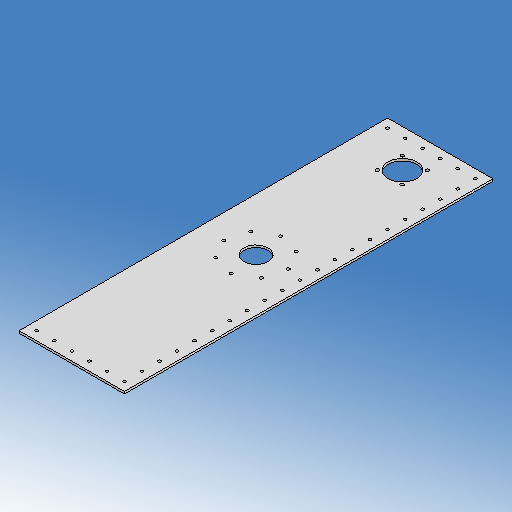
# Autodesk Inventor part: Armplate
Saved by Autodesk Inventor 2025 (Build 290162000, 162)
## iProperties
Created: 2024-06-23
Part Number: Armplate
Material: Generic
Document SubType Name: Modeling
Designer: seene
Density: 1 g/cm^3
Appearance: Default
Author: seene
Autodesk Inventor part; units mm, degrees
ref_plane "YZ Plane" through (0, 0, 0) normal (1, 0, 0) x (0, 1, 0)
ref_plane "XZ Plane" through (0, 0, 0) normal (0, 1, 0) x (-1, 0, 0)
ref_plane "XY Plane" through (0, 0, 0) normal (0, 0, 1) x (1, 0, 0)
sketch "Sketch1" plane through (0, 0, 0) normal (0, 1, 0) x (-1, 0, 0)
  line L0 (0, 0) -> (152.4, 0)
  line L1 (152.4, 0) -> (152.4, -533.4)
  line L2 (152.4, -533.4) -> (0, -533.4)
  line L3 (0, -533.4) -> (0, 0)
  circle A0 centre (76.2, -266.7) radius 47.25 construction
  circle A1 centre (76.2, -266.7) radius 41.5 construction
  circle A2 centre (76.2, -266.7) radius 17.5
  circle A3 centre (101.5192, -233.8186) radius 2.25
  circle A4 centre (70.8527, -225.5459) radius 2.25
  circle A5 centre (43.3186, -241.3808) radius 2.25
  circle A6 centre (35.0459, -272.0473) radius 2.25
  circle A7 centre (50.8808, -299.5814) radius 2.25
  circle A8 centre (81.5473, -307.8541) radius 2.25
  circle A9 centre (109.0814, -292.0192) radius 2.25
  circle A10 centre (117.3541, -261.3527) radius 2.25
  circle A11 centre (139.7, -12.7) radius 2.0701
  line L4 (152.4, -24.6076) -> (0, -26.1951) construction
  line L5 (152.4, -266.7) -> (0, -266.7) construction
  circle A12 centre (139.7, -520.7) radius 2.0701
  line L6 (152.4, -508.7924) -> (0, -507.2049) construction
  circle A13 centre (114.3, -12.7) radius 2.0701
  circle A14 centre (114.3, -520.7) radius 2.0701
  circle A15 centre (88.9, -12.7) radius 2.0701
  circle A16 centre (88.9, -520.7) radius 2.0701
  circle A17 centre (63.5, -12.7) radius 2.0701
  circle A18 centre (63.5, -520.7) radius 2.0701
  circle A19 centre (38.1, -12.7) radius 2.0701
  circle A20 centre (38.1, -520.7) radius 2.0701
  circle A21 centre (12.7, -12.7) radius 2.0701
  circle A22 centre (12.7, -520.7) radius 2.0701
  circle A23 centre (12.7, -38.1) radius 2.0701
  circle A24 centre (12.7, -63.5) radius 2.0701
  circle A25 centre (12.7, -88.9) radius 2.0701
  circle A26 centre (12.7, -114.3) radius 2.0701
  circle A27 centre (12.7, -139.7) radius 2.0701
  circle A28 centre (12.7, -165.1) radius 2.0701
  circle A29 centre (12.7, -190.5) radius 2.0701
  circle A30 centre (12.7, -215.9) radius 2.0701
  circle A31 centre (12.7, -241.3) radius 2.0701
  circle A32 centre (12.7, -266.7) radius 2.0701
  circle A33 centre (12.7, -292.1) radius 2.0701
  circle A34 centre (12.7, -317.5) radius 2.0701
  circle A35 centre (12.7, -342.9) radius 2.0701
  circle A36 centre (12.7, -368.3) radius 2.0701
  circle A37 centre (12.7, -393.7) radius 2.0701
  circle A38 centre (12.7, -419.1) radius 2.0701
  circle A39 centre (12.7, -444.5) radius 2.0701
  circle A40 centre (12.7, -469.9) radius 2.0701
  circle A41 centre (12.7, -495.3) radius 2.0701
  circle A42 centre (76.2, -478.7) radius 21
  circle A43 centre (76.2, -266.7) radius 212 construction
  circle A44 centre (76.2, -478.7) radius 25.674 construction
  circle A45 centre (94.321, -496.8875) radius 2.5
  circle A46 centre (94.3875, -460.579) radius 2.5
  circle A47 centre (58.079, -460.5125) radius 2.5
  circle A48 centre (58.0125, -496.821) radius 2.5
  point P0 (76.2, 0)
  dimension "d9" = 83
  dimension "d31" = 424
  dimension "d0" = 152.4
  dimension "d1" = 533.4
  dimension "d2" = 94.5
  dimension "d3" = 4.5
  dimension "d4" = 35
  dimension "d7" = 360
  dimension "d10" = 4.1402
  dimension "d11" = 25.4
  dimension "d12" = 12.7
  dimension "d13" = 12.7
  dimension "d16" = 25.4
  dimension "d23" = 25.4
  dimension "d30" = 42
  dimension "d32" = 5
  dimension "d35" = 360
  constraints: 46 centre point, 14 end point, 5 coincident, 4 midpoint, 3 symmetric about line, 2 horizontal, 2 parallel, 2 point on line, 2 vertical alignment, 1 perpendicular, 1 vertical, 93 other
  measures "d0" distance of L1.end L2.end
  measures "d1" distance of L0.end L1.end
  measures "d2" diameter of A0
  measures "d3" diameter of A3
  measures "d4" diameter of A2
  measures "d10" diameter of A11
  measures "d11" distance from line of L4 point (76.2, 0)
  measures "d12" distance from line of L1 A11.centre
  measures "d13" distance from line of A11.centre L0
  measures "d16" distance of A11.centre A13.centre
  measures "d23" distance of A21.centre A23.centre
  measures "d30" diameter of A42
  measures "d32" diameter of A45
extrude "Extrusion1" add sketch "Sketch1" along normal blind 3.175
body "Solid1"
